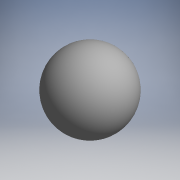
# Autodesk Inventor part: 51111 Ball
Saved by Autodesk Inventor 2023 (Build 270158000, 158)
## iProperties
Part Number: 51111 Ball
Material: 一般
Catalog Web Link: www.cadenas.de
Description: tb sdt b-
Vendor: NTN
Document SubType Name: Modeling
Designer: partserver
Manufacturer: NTN
Mass: 0.376637 g
Surface Area: 2.52212 cm^2
Volume: 0.376637 cm^3
Density: 1 g/cm^3
Appearance: PSOLRGB-192-192-192
Category: PARTsolutions
Company: NTN
PSOL_IDENT_0: {$CADENAS_DATA\23d-libs\ntn\ball_roller_bearings\thrust_b\tb_sdt_b.prj},165 {VTYP=3D},{NB=51111 Ball
PSOL_IDENT_1: },{LINA=51111 Ball},{NN=tb sdt b},{DATE=21.12.2021 04:23:12},{GEOMDATE=08.04.2020 13:28:36},{VERSION=
PSOL_IDENT_2: },{LINEID=11140},{WBVAR=},{WBNUMERIC=}  {NB=51111 Ball},{LINA=51111 Ball},{KT=DUMMY},{IDNR=},{SD=55}
PSOL_IDENT_3: ,{D=78},{T=16},{R=0.6},{ORDER=51111},{CA=35},{COA=93},{CAF=3 550},{COAF=9 500},{NG=2 800},{NO=4 000}
PSOL_IDENT_4: ,{D1=78},{SD1=57},{MASS=0.23},{DA1=69},{DA=64},{RAS=0,6},{X=10.50000},{BN=13.316964},{X1=11.50000},{
PSOL_IDENT_5: O=208.81},{T1=5.33333},{T2=5.33333},{RB=4.48000}
NB: 51111 Ball
NN: tb sdt b
NBSYN: $ORDER. Ball
LINA: 51111 Ball
CATALOG: NTN Corporation
SD: 55
D: 78
T: 16
R: 0.6
ORDER: 51111
CA: 35
COA: 93
CAF: 3 550
COAF: 9 500
NG: 2 800
NO: 4 000
D1: 78
SD1: 57
MASS: 0.23
DA1: 69
DA: 64
RAS: 0,6
SUPPLIER: NTN
ARTICLENO: 51111 Ball
BOMINFO: 51111 Ball
CREATOR: CADENAS GmbH
Title: 51111 Ball
Author: Cadenas PARTsolutions
Autodesk Inventor part; units mm, degrees
sketch "Sketch_1" plane through (0, 0, 0) normal (0, 0, 1) x (1, 0, 0)
  line L0 (4.48, 0) -> (-4.48, 0)
  arc A0 (4.48, 0) -> (-4.48, 0) centre (0, 0) ccw
  line L1 (4.48, 0) -> (-4.48, 0)
  constraints: 4 end point, 2 point on circle, 1 centre point
revolve "Revolution1" add sketch "Sketch_1" angle 360 about axis through (4.48, 0, 0) along (1, 0, 0)
ref_plane "tb_sdt_b_XY" through (0, 0, 0) normal (1, 0, 0) x (0, 0, -1)
ref_plane "tb_sdt_b_YZ" through (0, 0, 0) normal (0, 0, -1) x (0, 1, 0)
ref_plane "tb_sdt_b_ZX" through (0, 0, 0) normal (0, 1, 0) x (1, 0, 0)
body "Solid1"
